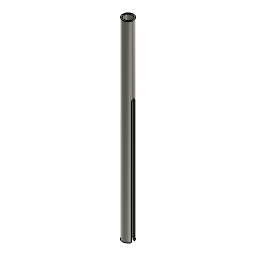
NAN tower v1 (Autodesk Fusion 360 design; units mm, degrees)
Autodesk Fusion 360 part; units mm, degrees
sketch "Sketch1" plane through (0, 0, 0) normal (0, 0, 1) x (1, 0, 0)
  circle A0 centre (0, 0) radius 3.9
  circle A1 centre (0, 0) radius 3
  dimension "d168" = 7.8
  dimension "d169" = 6
  constraint coincident A0.centre A1.centre
  constraint concentric A0 A1
  measures "d168" diameter of A0
  measures "d169" diameter of A1
extrude "Extrude1" add sketch "Sketch1" along normal blind 140
sketch "Sketch2" plane through (0, 0, 0) normal (1, 0, 0) x (0, 1, 0)
  line L0 (1.1, 0) -> (1.1, 89)
  arc A0 (1.1, 89) -> (-1.1, 89) centre (0, 89) ccw
  line L1 (-1.1, 89) -> (-1.1, 0)
  arc A1 (-1.1, 0) -> (1.1, 0) centre (0, 0) ccw
  line L2 (0, -1.1) -> (0, 90.1) construction
  line L3 (3.9, 0) -> (-3.9, 0)
  line L4 (3.9, 140) -> (-3.9, 140)
  line L5 (3.9, 0) -> (-3.9, 0)
  dimension "d172" = 2.2
  dimension "d174" = 89
  constraint tangent L0 A0
  constraint tangent A0 L1
  constraint parallel L0 L1
  constraint tangent L1 A1
  constraint tangent L0 A1
  constraint midpoint A1 L2.start
  constraint midpoint A0 L2.end
  constraint vertical L2
  constraint coincident A1.centre L5
  measures "d172" distance of L0 L1
  measures "d174" distance of A0.centre L3
extrude "Extrude2" cut sketch "Sketch2" along normal mid plane 20 contours L0 A0 L1 L3 L5
